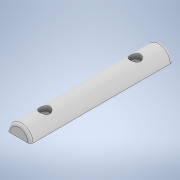
# Autodesk Inventor part: BodySiliconeRubber
Saved by Autodesk Inventor 2022.2 (Build 262287030, 287C)
## iProperties
Created: 2022-03-03
Part Number: BodySiliconeRubber
Material: Generic
Document SubType Name: Modeling
Designer: Jochen
Density: 1 g/cm^3
Appearance: Default
Author: Jochen
Autodesk Inventor part; units mm, degrees
ref_plane "YZ Plane" through (0, 0, 0) normal (1, 0, 0) x (0, 1, 0)
ref_plane "XZ Plane" through (0, 0, 0) normal (0, 1, 0) x (-1, 0, 0)
ref_plane "XY Plane" through (0, 0, 0) normal (0, 0, 1) x (1, 0, 0)
sketch "Sketch3" plane through (0, 0, 0) normal (0, 0, 1) x (1, 0, 0)
  line L0 (0, -1.8) -> (0, 10.8) construction
  line L1 (-12.6, 0) -> (12.6, 0) construction
  line L2 (-9, 0) -> (9, 0)
  line L3 (9, 0) -> (9, 0)
  arc A0 (9, 0) -> (-9, 0) centre (0, 0) ccw
  line L4 (-9, 0) -> (-9, 0)
  dimension "d20" = 18
  dimension "d21" = 0
  constraints: 6 end point, 2 point on circle, 2 point on line, 2 tangent, 1 centre point, 1 parallel, 1 vertical, 1 other
  measures "d20" distance between parallel lines of L3 L4
  measures "d21" distance of L2.end L3.end
extrude "Extrusion3" add sketch "Sketch3" along normal blind 110
fillet "Fillet1" radius 2 2 edges at (0, 9, 0) (0, 9, 110)
sketch "Sketch4" plane through (0, 0, 0) normal (0, 1, 0) x (-1, 0, 0)
  circle A0 centre (0, 90) radius 1.25
  circle A1 centre (0, 20) radius 1.25
  circle A2 centre (0, 20) radius 4
  circle A3 centre (0, 90) radius 4
  line L0 (9, 55) -> (-9, 55) construction
  arc A4 (-7, 110) -> (-9, 108) centre (-7, 108) ccw projected
  line L1 (-7, 110) -> (7, 110) projected
  arc A5 (9, 108) -> (7, 110) centre (7, 108) ccw projected
  line L2 (9, 108) -> (9, 2) projected
  arc A6 (7, 0) -> (9, 2) centre (7, 2) ccw projected
  line L3 (7, 0) -> (-7, 0) projected
  arc A7 (-9, 2) -> (-7, 0) centre (-7, 2) ccw projected
  line L4 (-9, 2) -> (-9, 108) projected
  point P0 (0, 0)
  dimension "d25" = 8
  dimension "d26" = 2.5
  dimension "d31" = 70
  constraints: 4 centre point, 2 coincident, 2 end point, 2 equal radius, 1 midpoint, 2 other
  measures "d25" diameter of A2
  measures "d26" diameter of A1
  measures "d31" distance of A1.centre A0.centre
extrude "Extrusion4" cut sketch "Sketch4" along normal blind 85 contours A0 | A1 | A2 | A3
extrude "Extrusion5" add sketch "Sketch4" along normal blind 5 from surface at 0 contours A2 | A3
body "Solid3"
